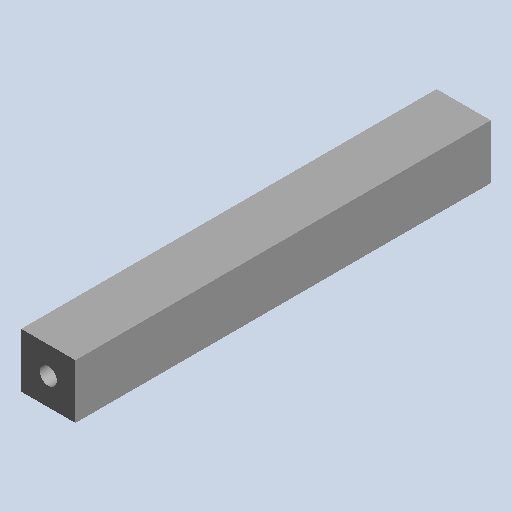
# Autodesk Inventor part: Frame_member
Saved by Autodesk Inventor 2026 (Build 300175050, 175E)
## iProperties
Part Number: Frame_member
Material: Generic
Document SubType Name: Modeling
Designer: Kartik
Mass: 56.4306 g
Surface Area: 160.058 cm^2
Volume: 56.4306 cm^3
Density: 1 g/cm^3
Appearance: Default
Author: Kartik
Autodesk Inventor part; units mm, degrees
ref_plane "YZ Plane" through (0, 0, 0) normal (1, 0, 0) x (0, 1, 0)
ref_plane "XZ Plane" through (0, 0, 0) normal (0, 1, 0) x (-1, 0, 0)
ref_plane "XY Plane" through (0, 0, 0) normal (0, 0, 1) x (1, 0, 0)
sketch "Sketch1" plane through (0, 0, 0) normal (0, 0, 1) x (1, 0, 0)
  line L0 (-7.2143, 7.8571) -> (12.7857, 7.8571)
  line L1 (12.7857, 7.8571) -> (12.7857, -12.1429)
  line L2 (12.7857, -12.1429) -> (-7.2143, -12.1429)
  line L3 (-7.2143, -12.1429) -> (-7.2143, 7.8571)
  point P0 (0, 0)
  dimension "d0" = 20
  dimension "d1" = 20
  constraints: 8 end point, 2 parallel, 1 horizontal, 1 perpendicular
  measures "d0" distance of L0.start L0.end
  measures "d1" distance of L2.end L0.start
extrude "Extrusion1" add sketch "Sketch1" along normal blind 153
sketch "Sketch2" plane through (0, 0, 153) normal (0, 0, 1) x (1, 0, 0)
  line L0 (12.7857, 7.8571) -> (-7.2143, 7.8571) projected
  line L1 (12.7857, -12.1429) -> (12.7857, 7.8571) projected
  point P0 (0, 0)
  point P1 (2.7857, -2.1429)
  dimension "d4" = 10
  dimension "d5" = 10
  measures "d4" distance from line of L0 point (2.786, -2.143)
  measures "d5" distance from line of L1 point (2.786, -2.143)
hole "Hole1" at (2.7857, -2.1429, 153) direction (0, 0, -1) diameter 6.3 end through all
body "Solid1"
